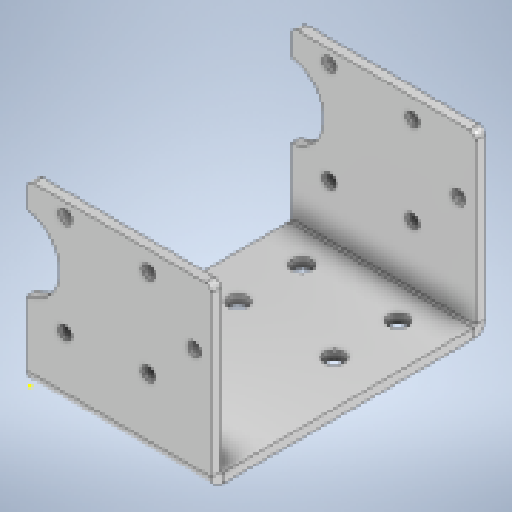
# Autodesk Inventor part: axis_16_bottom_frame
Saved by Autodesk Inventor 2026.1 (Build 301233000, 233)
## iProperties
Created: 2025-06-30
Part Number: axis_16_bottom_frame
Material: Aluminum 6061-AHC
Document SubType Name: Sheet Metal
Designer: LG
Density: 2.7 g/cm^3
Sheet Metal Rule: Default_mm
Appearance: Aluminum - Dark
Author: LG
Autodesk Inventor part; units mm, degrees
ref_plane "YZ Plane" through (0, 0, 0) normal (1, 0, 0) x (0, 1, 0)
ref_plane "XZ Plane" through (0, 0, 0) normal (0, 1, 0) x (-1, 0, 0)
ref_plane "XY Plane" through (0, 0, 0) normal (0, 0, 1) x (1, 0, 0)
sketch "Sketch1" plane through (0, 0, 0) normal (0, 1, 0) x (-1, 0, 0)
  line L0 (0.53, 20.25) -> (-28.77, 20.25)
  line L1 (-28.77, 20.25) -> (-28.77, -20.25)
  line L2 (-28.77, -20.25) -> (0.53, -20.25)
  line L3 (0.53, -20.25) -> (0.53, 20.25)
  point P0 (0, 0)
  dimension "d0" = 40.5
  dimension "d1" = 29.3
  dimension "d2" = -0.53
  dimension "d3" = 20.25
  measures "d0" distance of L2.end L0.start
  measures "d1" distance of L1.end L2.end
  measures "d2" distance from line of point (0, 0) L3
  measures "d3" distance from line of point (0, 0) L2
extrude "Plate1" add sketch "Sketch1" along normal blind 1.5
sketch "Sketch2" plane through (28.77, 0, 21.75) normal (0, 0, -1) x (-1, 0, 0)
  line L0 (29.3, 0) -> (0, 0)
  line L1 (0, 0) -> (0, 28.14)
  line L2 (0, 28.14) -> (29.3, 28.14)
  line L3 (29.3, 28.14) -> (29.3, 0)
  constraints: 8 end point
edge flange "Flange1" height 28.14 angle 90 thickness 1.5 bend radius 0.31 thickness toward (0, 0, -1) relief straight relief width 1.5 relief depth 0.75 corner gap 0.31 corner form 0 edges at (14.12, 1.5, 20.25) (14.12, 1.5, -20.25) wall of the first edge with corners at (-0.53, 0, 21.75) (28.77, 0, 21.75) (28.77, 28.14, 21.75) (-0.53, 28.14, 21.75)
bend "Bend1"
corner "Corner1"
sketch "Sketch6" plane through (-0.53, 28.14, 21.75) normal (0, 0, 1) x (1, 0, 0)
  point P0 (0.53, -28.14)
sketch "Sketch9" plane through (28.77, 28.14, -21.75) normal (0, 0, -1) x (-1, 0, 0)
  circle A0 centre (30.1, -10.07) radius 6
  point P0 (28.77, -28.14)
  constraints: 1 centre point, 2 other
extrude "Cut2" cut sketch "Sketch9" against normal blind 1.5
sketch "Sketch10" plane through (-0.53, 28.14, 21.75) normal (0, 0, 1) x (1, 0, 0)
  point P0 (0.53, -28.14)
sketch "Sketch11" plane through (-0.53, 28.14, 21.75) normal (0, 0, 1) x (1, 0, 0)
  point P0 (0.53, -28.14)
sketch "Sketch15" plane through (0, 0, 0) normal (0, -1, 0) x (1, 0, 0)
  point P0 (0, 0)
sketch "Sketch16" plane through (0, 0, 0) normal (0, -1, 0) x (1, 0, 0)
  circle A0 centre (6.47, -4.8) radius 1.55
  line L0 (28.77, 19.94) -> (-0.53, 19.94) projected
  line L1 (-0.53, -19.94) -> (-0.53, 19.94) projected
  circle A1 centre (21.77, -4.8) radius 1.55
  line L2 (28.77, 19.94) -> (28.77, -19.94) projected
  circle A2 centre (6.47, -14.94) radius 1.55
  circle A3 centre (21.77, -14.94) radius 1.55
  line L3 (-0.53, -19.94) -> (28.77, -19.94) projected
  point P0 (0, 0)
  dimension "d65" = 3.1
  dimension "d67" = 7
  dimension "d68" = 3.1
  dimension "d70" = 7
  dimension "d71" = 3.1
  dimension "d73" = 7
  dimension "d74" = 3.1
  dimension "d76" = 7
  dimension "d96" = 5
  dimension "d97" = 15.14
  dimension "d98" = 5
  dimension "d99" = 15.14
  constraints: 4 centre point
  measures "d65" diameter of A0
  measures "d67" distance from line of L1 A0.centre
  measures "d68" diameter of A1
  measures "d70" distance from line of L2 A1.centre
  measures "d71" diameter of A2
  measures "d73" distance from line of L1 A2.centre
  measures "d74" diameter of A3
  measures "d76" distance from line of L2 A3.centre
  measures "d96" distance from line of L3 A3.centre
  measures "d97" distance from line of L3 A1.centre
  measures "d98" distance from line of L3 A2.centre
  measures "d99" distance from line of L3 A0.centre
extrude "Cut6" cut sketch "Sketch16" against normal blind 1.5 contours A0 | A1 | A2 | A3
sketch "Sketch18" plane through (-0.53, 28.14, 21.75) normal (0, 0, 1) x (1, 0, 0)
  circle A0 centre (-0.8, -10.07) radius 6
  point P0 (0.53, -28.14)
  constraints: 1 centre point, 2 other
extrude "Cut7" cut sketch "Sketch18" against normal blind 1.5
fillet "Corner Round1" radius 1 4 edges at (28.77, 28.14, -21) (-0.53, 28.14, -21) (-0.53, 28.14, 21) (28.77, 28.14, 21)
sketch "Sketch21" plane through (28.77, 1.81, -21.75) normal (0, 0, -1) x (-1, 0, 0)
  circle A0 centre (2.68, 16.26) radius 0.7835 projected
  circle A1 centre (9.98, 23.26) radius 0.7835 projected
  circle A2 centre (23.2, 24.26) radius 0.7835 projected
  circle A3 centre (9.98, 9.26) radius 0.7835 projected
  circle A4 centre (23.2, 8.26) radius 0.7835 projected
  point P0 (28.77, -1.81)
hole "Hole8" at (18.79, 25.07, -21.75) at (5.57, 26.07, -21.75) at (26.09, 18.07, -21.75) at (18.79, 11.07, -21.75) at (5.57, 10.07, -21.75) direction (0, 0, 1) diameter 2.1 depth 1.5 tip angle 118
sketch "Sketch22" plane through (-0.53, 1.81, 21.75) normal (0, 0, 1) x (1, 0, 0)
  circle A0 centre (26.8, 23.785) radius 0.7835 projected
  circle A1 centre (11.7, 23.785) radius 0.7835 projected
  circle A2 centre (26.8, 8.735) radius 0.7835 projected
  circle A3 centre (11.7, 8.735) radius 0.7835 projected
  point P0 (0.53, -1.81)
hole "Hole9" at (11.17, 25.595, 21.75) at (11.17, 10.545, 21.75) at (26.27, 25.595, 21.75) at (26.27, 10.545, 21.75) direction (0, 0, -1) diameter 2.1 depth 1.5 tip angle 118
equation "\"d57\" = Thickness"
equation "\"d77\" = Thickness"
equation "\"d86\" = Thickness"
equation "\"d119\" = Thickness"
equation "\"d4\" = Thickness"
equation "\"d5\" = BendReliefWidth"
equation "\"d6\" = BendReliefDepth"
equation "\"d7\" = MinimumRemnant"
equation "\"d8\" = TransitionRadius"
equation "\"d11\" = BendRadius"
equation "\"d12\" = CornerReliefSize"
equation "\"d13\" = GapSize"
equation "\"d14\" = JacobiRadiusSize"
equation "\"BendReliefWidth\" = Thickness"
equation "\"BendReliefDepth\" = 0.5 * Thickness"
equation "\"CornerReliefSize\" = 4 * Thickness"
equation "\"MinimumRemnant\" = 2 * Thickness"
equation "\"TransitionRadius\" = BendRadius"
equation "\"JacobiRadiusSize\" = BendRadius"
equation "\"GapSize\" = Thickness"
equation "\"Thickness\" = 1.5"
equation "\"BendRadius\" = 0.31"
body "Solid1"
